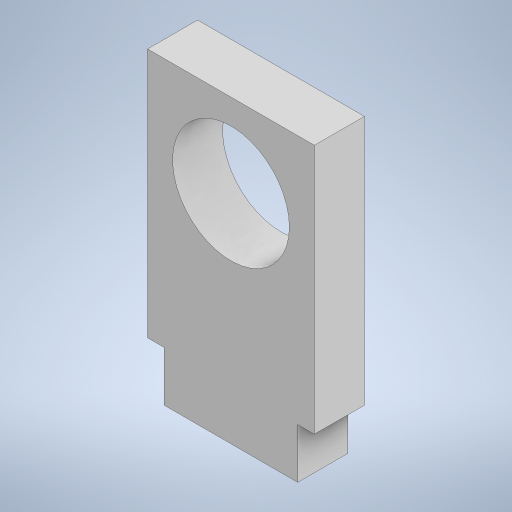
# Autodesk Inventor part: land
Saved by Autodesk Inventor 2023 (Build 270158000, 158)
## iProperties
Created: 2023-05-05
Part Number: land
Material: 一般
Document SubType Name: Modeling
Designer: 陳詩穎
Density: 1 g/cm^3
Appearance: 預設
Author: 陳詩穎
Autodesk Inventor part; units mm, degrees
ref_plane "YZ Plane" through (0, 0, 0) normal (1, 0, 0) x (0, 1, 0)
ref_plane "XZ Plane" through (0, 0, 0) normal (0, 1, 0) x (-1, 0, 0)
ref_plane "XY Plane" through (0, 0, 0) normal (0, 0, 1) x (1, 0, 0)
sketch "草圖1" plane through (0, 0, 0) normal (0, 0, 1) x (1, 0, 0)
  line L0 (-5, 15) -> (5, 15)
  line L1 (5, 15) -> (5, 0)
  line L2 (5, 0) -> (-5, 0)
  line L3 (-5, 0) -> (-5, 15)
  line L4 (-4, 0) -> (4, 0)
  line L5 (4, 0) -> (4, -3)
  line L6 (4, -3) -> (-4, -3)
  line L7 (-4, -3) -> (-4, 0)
  circle A0 centre (0, 10) radius 3.5
  point P0 (0, 0)
  point P1 (0, 0)
  dimension "d0" = 3
  dimension "d1" = 8
  dimension "d2" = 15
  dimension "d3" = 7
  dimension "d4" = 5
  dimension "d5" = 10
  constraints: 16 end point, 4 parallel, 2 horizontal, 2 midpoint, 2 perpendicular, 1 centre point, 1 coincident, 1 horizontal alignment, 1 point on line, 1 vertical alignment
  measures "d0" distance of L4.end L5.end
  measures "d1" distance of L5.end L6.end
  measures "d2" distance between parallel lines of L2 L0
  measures "d3" diameter of A0
  measures "d4" distance from line of A0.centre L0
  measures "d5" distance between parallel lines of L3 L1
extrude "擠出1" add sketch "草圖1" along normal blind 3
